Autodesk Fusion 360 part; units mm, degrees
(part 2 of 6)
  arc A437 (-116.0003, -83.2613) -> (-115.4978, -80.8724) centre (-117.2994, -81.7407) ccw
  arc A438 (-109.575, -88.7321) -> (-112.01, -88.5567) centre (-110.9063, -90.2247) ccw
  arc A439 (-112.6799, -88.4476) -> (-112.01, -88.5567) centre (-112.2859, -88.1398) ccw
  line L220 (-112.88, -88.1915) -> (-112.6799, -88.4476)
  line L221 (-112.88, -88.1915) -> (-113.08, -87.9354)
  arc A440 (-113.0239, -87.259) -> (-113.08, -87.9354) centre (-112.686, -87.6276) ccw
  arc A441 (-113.0239, -87.259) -> (-112.605, -84.8539) centre (-114.3753, -85.7846) ccw
  arc A442 (-106.4116, -92.5022) -> (-108.8511, -92.4119) centre (-107.6899, -94.0403) ccw
  arc A443 (-109.5244, -92.3262) -> (-108.8511, -92.4119) centre (-109.1414, -92.0048) ccw
  line L222 (-109.7334, -92.0772) -> (-109.5244, -92.3262)
  line L223 (-109.7334, -92.0772) -> (-109.9423, -91.8283)
  arc A444 (-109.9097, -91.1503) -> (-109.9423, -91.8283) centre (-109.5592, -91.5069) ccw
  arc A445 (-109.9097, -91.1503) -> (-109.575, -88.7321) centre (-111.3118, -89.724) ccw
  arc A446 (-103.1185, -96.1595) -> (-105.5597, -96.1544) centre (-104.3424, -97.7413) ccw
  arc A447 (-106.2356, -96.0923) -> (-105.5597, -96.1544) centre (-105.864, -95.7577) ccw
  line L224 (-106.4531, -95.8508) -> (-106.2356, -96.0923)
  line L225 (-106.4531, -95.8508) -> (-106.6705, -95.6092)
  arc A448 (-106.6617, -94.9306) -> (-106.6705, -95.6092) centre (-106.299, -95.2747) ccw
  arc A449 (-106.6617, -94.9306) -> (-106.4116, -92.5022) centre (-108.1126, -93.554) ccw
  arc A450 (-99.6997, -99.6997) -> (-102.1396, -99.7798) centre (-100.8677, -101.3233) ccw
  arc A451 (-102.8173, -99.7413) -> (-102.1396, -99.7798) centre (-102.4576, -99.394) ccw
  line L226 (-103.0431, -99.5075) -> (-102.8173, -99.7413)
  line L227 (-103.0431, -99.5075) -> (-103.2688, -99.2737)
  arc A452 (-103.2837, -98.5952) -> (-103.2688, -99.2737) centre (-102.9092, -98.9264) ccw
  arc A453 (-103.2837, -98.5952) -> (-103.1185, -96.1595) centre (-104.7818, -97.2701) ccw
  arc A454 (-96.1595, -103.1185) -> (-98.5952, -103.2837) centre (-97.2701, -104.7818) ccw
  arc A455 (-99.2737, -103.2688) -> (-98.5952, -103.2837) centre (-98.9264, -102.9092) ccw
  line L228 (-99.5075, -103.0431) -> (-99.2737, -103.2688)
  line L229 (-99.5075, -103.0431) -> (-99.7413, -102.8173)
  arc A456 (-99.7798, -102.1396) -> (-99.7413, -102.8173) centre (-99.394, -102.4576) ccw
  arc A457 (-99.7798, -102.1396) -> (-99.6997, -99.6997) centre (-101.3233, -100.8677) ccw
  arc A458 (-92.5022, -106.4116) -> (-94.9306, -106.6617) centre (-93.554, -108.1126) ccw
  arc A459 (-95.6092, -106.6705) -> (-94.9306, -106.6617) centre (-95.2747, -106.299) ccw
  line L230 (-95.8508, -106.4531) -> (-95.6092, -106.6705)
  line L231 (-95.8508, -106.4531) -> (-96.0923, -106.2356)
  arc A460 (-96.1544, -105.5597) -> (-96.0923, -106.2356) centre (-95.7577, -105.864) ccw
  arc A461 (-96.1544, -105.5597) -> (-96.1595, -103.1185) centre (-97.7413, -104.3424) ccw
  arc A462 (-88.7321, -109.575) -> (-91.1503, -109.9097) centre (-89.724, -111.3118) ccw
  arc A463 (-91.8283, -109.9423) -> (-91.1503, -109.9097) centre (-91.5069, -109.5592) ccw
  line L232 (-92.0772, -109.7334) -> (-91.8283, -109.9423)
  line L233 (-92.0772, -109.7334) -> (-92.3262, -109.5244)
  arc A464 (-92.4119, -108.8511) -> (-92.3262, -109.5244) centre (-92.0048, -109.1414) ccw
  arc A465 (-92.4119, -108.8511) -> (-92.5022, -106.4116) centre (-94.0403, -107.6899) ccw
  arc A466 (-84.8539, -112.605) -> (-87.259, -113.0239) centre (-85.7846, -114.3753) ccw
  arc A467 (-87.9354, -113.08) -> (-87.259, -113.0239) centre (-87.6276, -112.686) ccw
  line L234 (-88.1915, -112.88) -> (-87.9354, -113.08)
  line L235 (-88.1915, -112.88) -> (-88.4476, -112.6799)
  arc A468 (-88.5567, -112.01) -> (-88.4476, -112.6799) centre (-88.1398, -112.2859) ccw
  arc A469 (-88.5567, -112.01) -> (-88.7321, -109.575) centre (-90.2247, -110.9063) ccw
  arc A470 (-80.8724, -115.4978) -> (-83.2613, -116.0003) centre (-81.7407, -117.2994) ccw
  arc A471 (-83.9354, -116.0801) -> (-83.2613, -116.0003) centre (-83.6415, -115.6756) ccw
  line L236 (-84.1983, -115.889) -> (-83.9354, -116.0801)
  line L237 (-84.1983, -115.889) -> (-84.4612, -115.698)
  arc A472 (-84.5937, -115.0323) -> (-84.4612, -115.698) centre (-84.1673, -115.2935) ccw
  arc A473 (-84.5937, -115.0323) -> (-84.8539, -112.605) centre (-86.2991, -113.9875) ccw
  arc A474 (-76.7923, -118.2498) -> (-79.1623, -118.8354) centre (-77.5972, -120.0807) ccw
  arc A475 (-79.8331, -118.9387) -> (-79.1623, -118.8354) centre (-79.5535, -118.5241) ccw
  line L238 (-80.1025, -118.7569) -> (-79.8331, -118.9387)
  line L239 (-80.1025, -118.7569) -> (-80.372, -118.5752)
  arc A476 (-80.5276, -117.9145) -> (-80.372, -118.5752) centre (-80.0924, -118.1607) ccw
  arc A477 (-80.5276, -117.9145) -> (-80.8724, -115.4978) centre (-82.2684, -116.9299) ccw
  arc A478 (-72.6187, -120.8578) -> (-74.9667, -121.5258) centre (-73.3592, -122.7156) ccw
  arc A479 (-75.6336, -121.6523) -> (-74.9667, -121.5258) centre (-75.3686, -121.2283) ccw
  line L240 (-75.9092, -121.4801) -> (-75.6336, -121.6523)
  line L241 (-75.9092, -121.4801) -> (-76.1848, -121.3079)
  arc A480 (-76.3634, -120.653) -> (-76.1848, -121.3079) centre (-75.9199, -120.8839) ccw
  arc A481 (-76.3634, -120.653) -> (-76.7923, -118.2498) centre (-78.1375, -119.7298) ccw
  arc A482 (-68.3566, -123.3185) -> (-70.6799, -124.068) centre (-69.0318, -125.2011) ccw
  arc A483 (-71.3419, -124.2178) -> (-70.6799, -124.068) centre (-71.0919, -123.7848) ccw
  line L242 (-71.6234, -124.0553) -> (-71.3419, -124.2178)
  line L243 (-71.6234, -124.0553) -> (-71.9048, -123.8928)
  arc A484 (-72.1061, -123.2446) -> (-71.9048, -123.8928) centre (-71.6548, -123.4598) ccw
  arc A485 (-72.1061, -123.2446) -> (-72.6187, -120.8578) centre (-73.9114, -122.3838) ccw
  arc A486 (-64.0112, -125.629) -> (-66.3069, -126.4592) centre (-64.6203, -127.534) ccw
  arc A487 (-66.9633, -126.6319) -> (-66.3069, -126.4592) centre (-66.7286, -126.1905) ccw
  line L244 (-67.2503, -126.4793) -> (-66.9633, -126.6319)
  line L245 (-67.2503, -126.4793) -> (-67.5372, -126.3268)
  arc A488 (-67.761, -125.686) -> (-67.5372, -126.3268) centre (-67.3025, -125.8853) ccw
  arc A489 (-67.761, -125.686) -> (-68.3566, -123.3185) centre (-69.5953, -124.8887) ccw
  arc A490 (-59.5878, -127.7864) -> (-61.8532, -128.6962) centre (-60.13, -129.7115) ccw
  arc A491 (-62.5031, -128.8918) -> (-61.8532, -128.6962) centre (-62.2839, -128.4424) ccw
  line L246 (-62.7952, -128.7493) -> (-62.5031, -128.8918)
  line L247 (-62.7952, -128.7493) -> (-63.0873, -128.6068)
  arc A492 (-63.3334, -127.9742) -> (-63.0873, -128.6068) centre (-62.8682, -128.1574) ccw
  arc A493 (-63.3334, -127.9742) -> (-64.0112, -125.629) centre (-65.1943, -127.2415) ccw
  arc A494 (-55.0918, -129.7882) -> (-57.324, -130.7764) centre (-55.5665, -131.731) ccw
  arc A495 (-57.9668, -130.9946) -> (-57.324, -130.7764) centre (-57.7634, -130.5378) ccw
  line L248 (-58.2637, -130.8624) -> (-57.9668, -130.9946)
  line L249 (-58.2637, -130.8624) -> (-58.5606, -130.7302)
  arc A496 (-58.8286, -130.1066) -> (-58.5606, -130.7302) centre (-58.3572, -130.2734) ccw
  arc A497 (-58.8286, -130.1066) -> (-59.5878, -127.7864) centre (-60.7139, -129.4392) ccw
  arc A498 (-50.5287, -131.6318) -> (-52.7251, -132.6974) centre (-50.9353, -133.59) ccw
  arc A499 (-53.3598, -132.9378) -> (-52.7251, -132.6974) centre (-53.1725, -132.4742) ccw
  line L250 (-53.6612, -132.816) -> (-53.3598, -132.9378)
  line L251 (-53.6612, -132.816) -> (-53.9625, -132.6943)
  arc A500 (-54.2521, -132.0804) -> (-53.9625, -132.6943) centre (-53.7752, -132.2307) ccw
  arc A501 (-54.2521, -132.0804) -> (-55.0918, -129.7882) centre (-56.1596, -131.4793) ccw
  arc A502 (-45.904, -133.315) -> (-48.0619, -134.4566) centre (-46.2421, -135.2862) ccw
  arc A503 (-48.6879, -134.719) -> (-48.0619, -134.4566) centre (-48.5169, -134.2492) ccw
  line L252 (-48.9933, -134.6079) -> (-48.6879, -134.719)
  line L253 (-48.9933, -134.6079) -> (-49.2987, -134.4967)
  arc A504 (-49.6095, -133.8933) -> (-49.2987, -134.4967) centre (-49.1277, -134.0269) ccw
  arc A505 (-49.6095, -133.8933) -> (-50.5287, -131.6318) centre (-51.5368, -133.3591) ccw
  arc A506 (-41.2235, -134.8358) -> (-43.3402, -136.052) centre (-41.4925, -136.8177) ccw
  arc A507 (-43.9566, -136.3362) -> (-43.3402, -136.052) centre (-43.8021, -135.8606) ccw
  line L254 (-44.2657, -136.2357) -> (-43.9566, -136.3362)
  line L255 (-44.2657, -136.2357) -> (-44.5748, -136.1353)
  arc A508 (-44.9065, -135.5431) -> (-44.5748, -136.1353) centre (-44.4203, -135.6598) ccw
  arc A509 (-44.9065, -135.5431) -> (-45.904, -133.315) centre (-46.8513, -135.0765) ccw
  arc A510 (-36.4926, -136.1924) -> (-38.5656, -137.4817) centre (-36.6924, -138.1824) ccw
  arc A511 (-39.1717, -137.7872) -> (-38.5656, -137.4817) centre (-39.0339, -137.3065) ccw
  line L256 (-39.4841, -137.6976) -> (-39.1717, -137.7872)
  line L257 (-39.4841, -137.6976) -> (-39.7966, -137.608)
  arc A512 (-40.1487, -137.0278) -> (-39.7966, -137.608) centre (-39.6587, -137.1274) ccw
  arc A513 (-40.1487, -137.0278) -> (-41.2235, -134.8358) centre (-42.1086, -136.6293) ccw
  arc A514 (-31.7174, -137.383) -> (-33.7441, -138.7439) centre (-31.8475, -139.3787) ccw
  arc A515 (-34.3392, -139.0703) -> (-33.7441, -138.7439) centre (-34.2182, -138.5852) ccw
  line L258 (-34.6545, -138.9917) -> (-34.3392, -139.0703)
  line L259 (-34.6545, -138.9917) -> (-34.9699, -138.9131)
  arc A516 (-35.3421, -138.3455) -> (-34.9699, -138.9131) centre (-34.8489, -138.4279) ccw
  arc A517 (-35.3421, -138.3455) -> (-36.4926, -136.1924) centre (-37.3147, -138.0156) ccw
  arc A518 (-26.9034, -138.4062) -> (-28.8814, -139.837) centre (-26.9639, -140.4053) ccw
  arc A519 (-29.4648, -140.184) -> (-28.8814, -139.837) centre (-29.3608, -139.6949) ccw
  line L260 (-29.7827, -140.1164) -> (-29.4648, -140.184)
  line L261 (-29.7827, -140.1164) -> (-30.1006, -140.0489)
  arc A520 (-30.4923, -139.4946) -> (-30.1006, -140.0489) centre (-29.9966, -139.5598) ccw
  arc A521 (-30.4923, -139.4946) -> (-31.7174, -137.383) centre (-32.4753, -139.2338) ccw
  arc A522 (-22.0567, -139.2608) -> (-23.9836, -140.7598) centre (-22.0474, -141.2608) ccw
  arc A523 (-24.5545, -141.1269) -> (-23.9836, -140.7598) centre (-24.4676, -140.6345) ccw
  line L262 (-24.8745, -141.0705) -> (-24.5545, -141.1269)
  line L263 (-24.8745, -141.0705) -> (-25.1946, -141.014)
  arc A524 (-25.6055, -140.4738) -> (-25.1946, -141.014) centre (-25.1078, -140.5216) ccw
  arc A525 (-25.6055, -140.4738) -> (-26.9034, -138.4062) centre (-27.5963, -140.2824) ccw
  arc A526 (-17.1832, -139.9458) -> (-19.0565, -141.511) centre (-17.104, -141.9442) ccw
  arc A527 (-19.6143, -141.8979) -> (-19.0565, -141.511) centre (-19.5447, -141.4028) ccw
  line L264 (-19.9361, -141.8527) -> (-19.6143, -141.8979)
  line L265 (-19.9361, -141.8527) -> (-20.2579, -141.8074)
  arc A528 (-20.6874, -141.2818) -> (-20.2579, -141.8074) centre (-20.1883, -141.3123) ccw
  arc A529 (-20.6874, -141.2818) -> (-22.0567, -139.2608) centre (-22.6837, -141.16) ccw
  arc A530 (-12.2887, -140.4602) -> (-14.1063, -142.0899) centre (-12.1398, -142.4546) ccw
  arc A531 (-14.6501, -142.496) -> (-14.1063, -142.0899) centre (-14.5979, -141.9987) ccw
  line L266 (-14.9734, -142.462) -> (-14.6501, -142.496)
  line L267 (-14.9734, -142.462) -> (-15.2966, -142.428)
  arc A532 (-15.7441, -141.9177) -> (-15.2966, -142.428) centre (-15.2443, -141.9308) ccw
  arc A533 (-15.7441, -141.9177) -> (-17.1832, -139.9458) centre (-17.7435, -141.8657) ccw
  arc A534 (-7.3792, -140.8035) -> (-9.1388, -142.4956) centre (-7.1608, -142.7915) ccw
  arc A535 (-9.6682, -142.9205) -> (-9.1388, -142.4956) centre (-9.6333, -142.4217) ccw
  line L268 (-9.9924, -142.8978) -> (-9.6682, -142.9205)
  line L269 (-9.9924, -142.8978) -> (-10.3166, -142.8751)
  arc A536 (-10.7817, -142.3808) -> (-10.3166, -142.8751) centre (-10.2817, -142.3763) ccw
  arc A537 (-10.7817, -142.3808) -> (-12.2887, -140.4602) centre (-12.7816, -142.3985) ccw
  arc A538 (-2.4607, -140.9752) -> (-4.1602, -142.7278) centre (-2.1731, -142.9545) ccw
  arc A539 (-4.6744, -143.1708) -> (-4.1602, -142.7278) centre (-4.657, -142.6711) ccw
  line L270 (-4.9992, -143.1595) -> (-4.6744, -143.1708)
  line L271 (-4.9992, -143.1595) -> (-5.324, -143.1481)
  arc A540 (-5.8061, -142.6703) -> (-5.324, -143.1481) centre (-5.3066, -142.6484) ccw
  arc A541 (-5.8061, -142.6703) -> (-7.3792, -140.8035) centre (-7.8042, -142.7578) ccw
  arc A542 (2.4607, -140.9752) -> (0.8235, -142.786) centre (2.8173, -142.9432) ccw
  arc A543 (0.325, -143.2467) -> (0.8235, -142.786) centre (0.325, -142.7467) ccw
  line L272 (0, -143.2467) -> (0.325, -143.2467)
  line L273 (0, -143.2467) -> (-0.325, -143.2467)
  arc A544 (-0.8235, -142.786) -> (-0.325, -143.2467) centre (-0.325, -142.7467) ccw
  arc A545 (-0.8235, -142.786) -> (-2.4607, -140.9752) centre (-2.8173, -142.9432) ccw
  arc A546 (7.3792, -140.8035) -> (5.8061, -142.6703) centre (7.8042, -142.7578) ccw
  arc A547 (5.324, -143.1481) -> (5.8061, -142.6703) centre (5.3066, -142.6484) ccw
  line L274 (4.9992, -143.1595) -> (5.324, -143.1481)
  line L275 (4.9992, -143.1595) -> (4.6744, -143.1708)
  arc A548 (4.1602, -142.7278) -> (4.6744, -143.1708) centre (4.657, -142.6711) ccw
  arc A549 (4.1602, -142.7278) -> (2.4607, -140.9752) centre (2.1731, -142.9545) ccw
  arc A550 (12.2887, -140.4602) -> (10.7817, -142.3808) centre (12.7816, -142.3985) ccw
  arc A551 (10.3166, -142.8751) -> (10.7817, -142.3808) centre (10.2817, -142.3763) ccw
  line L276 (9.9924, -142.8978) -> (10.3166, -142.8751)
  line L277 (9.9924, -142.8978) -> (9.6682, -142.9205)
  arc A552 (9.1388, -142.4956) -> (9.6682, -142.9205) centre (9.6333, -142.4217) ccw
  arc A553 (9.1388, -142.4956) -> (7.3792, -140.8035) centre (7.1608, -142.7915) ccw
  arc A554 (17.1832, -139.9458) -> (15.7441, -141.9177) centre (17.7435, -141.8657) ccw
  arc A555 (15.2966, -142.428) -> (15.7441, -141.9177) centre (15.2443, -141.9308) ccw
  line L278 (14.9734, -142.462) -> (15.2966, -142.428)
  line L279 (14.9734, -142.462) -> (14.6501, -142.496)
  arc A556 (14.1063, -142.0899) -> (14.6501, -142.496) centre (14.5979, -141.9987) ccw
  arc A557 (14.1063, -142.0899) -> (12.2887, -140.4602) centre (12.1398, -142.4546) ccw
  arc A558 (22.0567, -139.2608) -> (20.6874, -141.2818) centre (22.6837, -141.16) ccw
  arc A559 (20.2579, -141.8074) -> (20.6874, -141.2818) centre (20.1883, -141.3123) ccw
  line L280 (19.9361, -141.8527) -> (20.2579, -141.8074)
  line L281 (19.9361, -141.8527) -> (19.6143, -141.8979)
  arc A560 (19.0565, -141.511) -> (19.6143, -141.8979) centre (19.5447, -141.4028) ccw
  arc A561 (19.0565, -141.511) -> (17.1832, -139.9458) centre (17.104, -141.9442) ccw
  arc A562 (26.9034, -138.4062) -> (25.6055, -140.4738) centre (27.5963, -140.2824) ccw
  arc A563 (25.1946, -141.014) -> (25.6055, -140.4738) centre (25.1078, -140.5216) ccw
  line L282 (24.8745, -141.0705) -> (25.1946, -141.014)
  line L283 (24.8745, -141.0705) -> (24.5545, -141.1269)
  arc A564 (23.9836, -140.7598) -> (24.5545, -141.1269) centre (24.4676, -140.6345) ccw
  arc A565 (23.9836, -140.7598) -> (22.0567, -139.2608) centre (22.0474, -141.2608) ccw
  arc A566 (31.7174, -137.383) -> (30.4923, -139.4946) centre (32.4753, -139.2338) ccw
  arc A567 (30.1006, -140.0489) -> (30.4923, -139.4946) centre (29.9966, -139.5598) ccw
  line L284 (29.7827, -140.1164) -> (30.1006, -140.0489)
  line L285 (29.7827, -140.1164) -> (29.4648, -140.184)
  arc A568 (28.8814, -139.837) -> (29.4648, -140.184) centre (29.3608, -139.6949) ccw
  arc A569 (28.8814, -139.837) -> (26.9034, -138.4062) centre (26.9639, -140.4053) ccw
  arc A570 (36.4926, -136.1924) -> (35.3421, -138.3455) centre (37.3147, -138.0156) ccw
  arc A571 (34.9699, -138.9131) -> (35.3421, -138.3455) centre (34.8489, -138.4279) ccw
  line L286 (34.6545, -138.9917) -> (34.9699, -138.9131)
  line L287 (34.6545, -138.9917) -> (34.3392, -139.0703)
  arc A572 (33.7441, -138.7439) -> (34.3392, -139.0703) centre (34.2182, -138.5852) ccw
  arc A573 (33.7441, -138.7439) -> (31.7174, -137.383) centre (31.8475, -139.3787) ccw
  arc A574 (41.2235, -134.8358) -> (40.1487, -137.0278) centre (42.1086, -136.6293) ccw
  arc A575 (39.7966, -137.608) -> (40.1487, -137.0278) centre (39.6587, -137.1274) ccw
  line L288 (39.4841, -137.6976) -> (39.7966, -137.608)
  line L289 (39.4841, -137.6976) -> (39.1717, -137.7872)
  arc A576 (38.5656, -137.4817) -> (39.1717, -137.7872) centre (39.0339, -137.3065) ccw
  arc A577 (38.5656, -137.4817) -> (36.4926, -136.1924) centre (36.6924, -138.1824) ccw
  arc A578 (45.904, -133.315) -> (44.9065, -135.5431) centre (46.8513, -135.0765) ccw
  arc A579 (44.5748, -136.1353) -> (44.9065, -135.5431) centre (44.4203, -135.6598) ccw
  line L290 (44.2657, -136.2357) -> (44.5748, -136.1353)
  line L291 (44.2657, -136.2357) -> (43.9566, -136.3362)
  arc A580 (43.3402, -136.052) -> (43.9566, -136.3362) centre (43.8021, -135.8606) ccw
  arc A581 (43.3402, -136.052) -> (41.2235, -134.8358) centre (41.4925, -136.8177) ccw
  arc A582 (50.5287, -131.6318) -> (49.6095, -133.8933) centre (51.5368, -133.3591) ccw
  arc A583 (49.2987, -134.4967) -> (49.6095, -133.8933) centre (49.1277, -134.0269) ccw
  line L292 (48.9933, -134.6079) -> (49.2987, -134.4967)
  line L293 (48.9933, -134.6079) -> (48.6879, -134.719)
  arc A584 (48.0619, -134.4566) -> (48.6879, -134.719) centre (48.5169, -134.2492) ccw
  arc A585 (48.0619, -134.4566) -> (45.904, -133.315) centre (46.2421, -135.2862) ccw
  arc A586 (55.0918, -129.7882) -> (54.2521, -132.0804) centre (56.1596, -131.4793) ccw
  arc A587 (53.9625, -132.6943) -> (54.2521, -132.0804) centre (53.7752, -132.2307) ccw
  line L294 (53.6612, -132.816) -> (53.9625, -132.6943)
  line L295 (53.6612, -132.816) -> (53.3598, -132.9378)
  arc A588 (52.7251, -132.6974) -> (53.3598, -132.9378) centre (53.1725, -132.4742) ccw
  arc A589 (52.7251, -132.6974) -> (50.5287, -131.6318) centre (50.9353, -133.59) ccw
  arc A590 (59.5878, -127.7864) -> (58.8286, -130.1066) centre (60.7139, -129.4392) ccw
  arc A591 (58.5606, -130.7302) -> (58.8286, -130.1066) centre (58.3572, -130.2734) ccw
  line L296 (58.2637, -130.8624) -> (58.5606, -130.7302)
  line L297 (58.2637, -130.8624) -> (57.9668, -130.9946)
  arc A592 (57.324, -130.7764) -> (57.9668, -130.9946) centre (57.7634, -130.5378) ccw
  arc A593 (57.324, -130.7764) -> (55.0918, -129.7882) centre (55.5665, -131.731) ccw
  arc A594 (64.0112, -125.629) -> (63.3334, -127.9742) centre (65.1943, -127.2415) ccw
  arc A595 (63.0873, -128.6068) -> (63.3334, -127.9742) centre (62.8682, -128.1574) ccw
  line L298 (62.7952, -128.7493) -> (63.0873, -128.6068)
  line L299 (62.7952, -128.7493) -> (62.5031, -128.8918)
  arc A596 (61.8532, -128.6962) -> (62.5031, -128.8918) centre (62.2839, -128.4424) ccw
  arc A597 (61.8532, -128.6962) -> (59.5878, -127.7864) centre (60.13, -129.7115) ccw
  arc A598 (68.3566, -123.3185) -> (67.761, -125.686) centre (69.5953, -124.8887) ccw
  arc A599 (67.5372, -126.3268) -> (67.761, -125.686) centre (67.3025, -125.8853) ccw
  line L300 (67.2503, -126.4793) -> (67.5372, -126.3268)
  line L301 (67.2503, -126.4793) -> (66.9633, -126.6319)
  arc A600 (66.3069, -126.4592) -> (66.9633, -126.6319) centre (66.7286, -126.1905) ccw
  arc A601 (66.3069, -126.4592) -> (64.0112, -125.629) centre (64.6203, -127.534) ccw
  arc A602 (72.6187, -120.8578) -> (72.1061, -123.2446) centre (73.9114, -122.3838) ccw
  arc A603 (71.9048, -123.8928) -> (72.1061, -123.2446) centre (71.6548, -123.4598) ccw
  line L302 (71.6234, -124.0553) -> (71.9048, -123.8928)
  line L303 (71.6234, -124.0553) -> (71.3419, -124.2178)
  arc A604 (70.6799, -124.068) -> (71.3419, -124.2178) centre (71.0919, -123.7848) ccw
  arc A605 (70.6799, -124.068) -> (68.3566, -123.3185) centre (69.0318, -125.2011) ccw
  arc A606 (76.7923, -118.2498) -> (76.3634, -120.653) centre (78.1375, -119.7298) ccw
  arc A607 (76.1848, -121.3079) -> (76.3634, -120.653) centre (75.9199, -120.8839) ccw
  line L304 (75.9092, -121.4801) -> (76.1848, -121.3079)
  line L305 (75.9092, -121.4801) -> (75.6336, -121.6523)
  arc A608 (74.9667, -121.5258) -> (75.6336, -121.6523) centre (75.3686, -121.2283) ccw
  arc A609 (74.9667, -121.5258) -> (72.6187, -120.8578) centre (73.3592, -122.7156) ccw
  arc A610 (80.8724, -115.4978) -> (80.5276, -117.9145) centre (82.2684, -116.9299) ccw
  arc A611 (80.372, -118.5752) -> (80.5276, -117.9145) centre (80.0924, -118.1607) ccw
  line L306 (80.1025, -118.7569) -> (80.372, -118.5752)
  line L307 (80.1025, -118.7569) -> (79.8331, -118.9387)
  arc A612 (79.1623, -118.8354) -> (79.8331, -118.9387) centre (79.5535, -118.5241) ccw
  arc A613 (79.1623, -118.8354) -> (76.7923, -118.2498) centre (77.5972, -120.0807) ccw
  arc A614 (84.8539, -112.605) -> (84.5937, -115.0323) centre (86.2991, -113.9875) ccw
  arc A615 (84.4612, -115.698) -> (84.5937, -115.0323) centre (84.1673, -115.2935) ccw
  line L308 (84.1983, -115.889) -> (84.4612, -115.698)
  line L309 (84.1983, -115.889) -> (83.9354, -116.0801)
  arc A616 (83.2613, -116.0003) -> (83.9354, -116.0801) centre (83.6415, -115.6756) ccw
  arc A617 (83.2613, -116.0003) -> (80.8724, -115.4978) centre (81.7407, -117.2994) ccw
  arc A618 (88.7321, -109.575) -> (88.5567, -112.01) centre (90.2247, -110.9063) ccw
  arc A619 (88.4476, -112.6799) -> (88.5567, -112.01) centre (88.1398, -112.2859) ccw
  line L310 (88.1915, -112.88) -> (88.4476, -112.6799)
  line L311 (88.1915, -112.88) -> (87.9354, -113.08)
  arc A620 (87.259, -113.0239) -> (87.9354, -113.08) centre (87.6276, -112.686) ccw
  arc A621 (87.259, -113.0239) -> (84.8539, -112.605) centre (85.7846, -114.3753) ccw
  arc A622 (92.5022, -106.4116) -> (92.4119, -108.8511) centre (94.0403, -107.6899) ccw
  arc A623 (92.3262, -109.5244) -> (92.4119, -108.8511) centre (92.0048, -109.1414) ccw
  line L312 (92.0772, -109.7334) -> (92.3262, -109.5244)
  line L313 (92.0772, -109.7334) -> (91.8283, -109.9423)
  arc A624 (91.1503, -109.9097) -> (91.8283, -109.9423) centre (91.5069, -109.5592) ccw
  arc A625 (91.1503, -109.9097) -> (88.7321, -109.575) centre (89.724, -111.3118) ccw
  arc A626 (96.1595, -103.1185) -> (96.1544, -105.5597) centre (97.7413, -104.3424) ccw
  arc A627 (96.0923, -106.2356) -> (96.1544, -105.5597) centre (95.7577, -105.864) ccw
  line L314 (95.8508, -106.4531) -> (96.0923, -106.2356)
  line L315 (95.8508, -106.4531) -> (95.6092, -106.6705)
  arc A628 (94.9306, -106.6617) -> (95.6092, -106.6705) centre (95.2747, -106.299) ccw
  arc A629 (94.9306, -106.6617) -> (92.5022, -106.4116) centre (93.554, -108.1126) ccw
  arc A630 (99.6997, -99.6997) -> (99.7798, -102.1396) centre (101.3233, -100.8677) ccw
  arc A631 (99.7413, -102.8173) -> (99.7798, -102.1396) centre (99.394, -102.4576) ccw
  line L316 (99.5075, -103.0431) -> (99.7413, -102.8173)
  line L317 (99.5075, -103.0431) -> (99.2737, -103.2688)
  arc A632 (98.5952, -103.2837) -> (99.2737, -103.2688) centre (98.9264, -102.9092) ccw
  arc A633 (98.5952, -103.2837) -> (96.1595, -103.1185) centre (97.2701, -104.7818) ccw
  arc A634 (103.1185, -96.1595) -> (103.2837, -98.5952) centre (104.7818, -97.2701) ccw
  arc A635 (103.2688, -99.2737) -> (103.2837, -98.5952) centre (102.9092, -98.9264) ccw
  line L318 (103.0431, -99.5075) -> (103.2688, -99.2737)
  line L319 (103.0431, -99.5075) -> (102.8173, -99.7413)
  arc A636 (102.1396, -99.7798) -> (102.8173, -99.7413) centre (102.4576, -99.394) ccw
  arc A637 (102.1396, -99.7798) -> (99.6997, -99.6997) centre (100.8677, -101.3233) ccw
  arc A638 (106.4116, -92.5022) -> (106.6617, -94.9306) centre (108.1126, -93.554) ccw
  arc A639 (106.6705, -95.6092) -> (106.6617, -94.9306) centre (106.299, -95.2747) ccw
  line L320 (106.4531, -95.8508) -> (106.6705, -95.6092)
  line L321 (106.4531, -95.8508) -> (106.2356, -96.0923)
  arc A640 (105.5597, -96.1544) -> (106.2356, -96.0923) centre (105.864, -95.7577) ccw
  arc A641 (105.5597, -96.1544) -> (103.1185, -96.1595) centre (104.3424, -97.7413) ccw
  arc A642 (109.575, -88.7321) -> (109.9097, -91.1503) centre (111.3118, -89.724) ccw
  arc A643 (109.9423, -91.8283) -> (109.9097, -91.1503) centre (109.5592, -91.5069) ccw
  line L322 (109.7334, -92.0772) -> (109.9423, -91.8283)
  line L323 (109.7334, -92.0772) -> (109.5244, -92.3262)
  arc A644 (108.8511, -92.4119) -> (109.5244, -92.3262) centre (109.1414, -92.0048) ccw
  arc A645 (108.8511, -92.4119) -> (106.4116, -92.5022) centre (107.6899, -94.0403) ccw
  arc A646 (112.605, -84.8539) -> (113.0239, -87.259) centre (114.3753, -85.7846) ccw
  arc A647 (113.08, -87.9354) -> (113.0239, -87.259) centre (112.686, -87.6276) ccw
  line L324 (112.88, -88.1915) -> (113.08, -87.9354)
  line L325 (112.88, -88.1915) -> (112.6799, -88.4476)
  arc A648 (112.01, -88.5567) -> (112.6799, -88.4476) centre (112.2859, -88.1398) ccw
  arc A649 (112.01, -88.5567) -> (109.575, -88.7321) centre (110.9063, -90.2247) ccw
  arc A650 (115.4978, -80.8724) -> (116.0003, -83.2613) centre (117.2994, -81.7407) ccw
  arc A651 (116.0801, -83.9354) -> (116.0003, -83.2613) centre (115.6756, -83.6415) ccw
  line L326 (115.889, -84.1983) -> (116.0801, -83.9354)
  line L327 (115.889, -84.1983) -> (115.698, -84.4612)
  arc A652 (115.0323, -84.5937) -> (115.698, -84.4612) centre (115.2935, -84.1673) ccw
  arc A653 (115.0323, -84.5937) -> (112.605, -84.8539) centre (113.9875, -86.2991) ccw
  arc A654 (118.2498, -76.7923) -> (118.8354, -79.1623) centre (120.0807, -77.5972) ccw
  arc A655 (118.9387, -79.8331) -> (118.8354, -79.1623) centre (118.5241, -79.5535) ccw
  line L328 (118.7569, -80.1025) -> (118.9387, -79.8331)
  line L329 (118.7569, -80.1025) -> (118.5752, -80.372)
  arc A656 (117.9145, -80.5276) -> (118.5752, -80.372) centre (118.1607, -80.0924) ccw
  arc A657 (117.9145, -80.5276) -> (115.4978, -80.8724) centre (116.9299, -82.2684) ccw
  arc A658 (120.8578, -72.6187) -> (121.5258, -74.9667) centre (122.7156, -73.3592) ccw
  arc A659 (121.6523, -75.6336) -> (121.5258, -74.9667) centre (121.2283, -75.3686) ccw
  line L330 (121.4801, -75.9092) -> (121.6523, -75.6336)
  line L331 (121.4801, -75.9092) -> (121.3079, -76.1848)
  arc A660 (120.653, -76.3634) -> (121.3079, -76.1848) centre (120.8839, -75.9199) ccw
  arc A661 (120.653, -76.3634) -> (118.2498, -76.7923) centre (119.7298, -78.1375) ccw
  arc A662 (123.3185, -68.3566) -> (124.068, -70.6799) centre (125.2011, -69.0318) ccw
  arc A663 (124.2178, -71.3419) -> (124.068, -70.6799) centre (123.7848, -71.0919) ccw
  line L332 (124.0553, -71.6234) -> (124.2178, -71.3419)
  line L333 (124.0553, -71.6234) -> (123.8928, -71.9048)
  arc A664 (123.2446, -72.1061) -> (123.8928, -71.9048) centre (123.4598, -71.6548) ccw
  arc A665 (123.2446, -72.1061) -> (120.8578, -72.6187) centre (122.3838, -73.9114) ccw
  arc A666 (125.629, -64.0112) -> (126.4592, -66.3069) centre (127.534, -64.6203) ccw
  arc A667 (126.6319, -66.9633) -> (126.4592, -66.3069) centre (126.1905, -66.7286) ccw
  line L334 (126.4793, -67.2503) -> (126.6319, -66.9633)
  line L335 (126.4793, -67.2503) -> (126.3268, -67.5372)
  arc A668 (125.686, -67.761) -> (126.3268, -67.5372) centre (125.8853, -67.3025) ccw
  arc A669 (125.686, -67.761) -> (123.3185, -68.3566) centre (124.8887, -69.5953) ccw
  arc A670 (127.7864, -59.5878) -> (128.6962, -61.8532) centre (129.7115, -60.13) ccw
  arc A671 (128.8918, -62.5031) -> (128.6962, -61.8532) centre (128.4424, -62.2839) ccw
  line L336 (128.7493, -62.7952) -> (128.8918, -62.5031)
  line L337 (128.7493, -62.7952) -> (128.6068, -63.0873)
  arc A672 (127.9742, -63.3334) -> (128.6068, -63.0873) centre (128.1574, -62.8682) ccw
  arc A673 (127.9742, -63.3334) -> (125.629, -64.0112) centre (127.2415, -65.1943) ccw
  arc A674 (129.7882, -55.0918) -> (130.7764, -57.324) centre (131.731, -55.5665) ccw
  arc A675 (130.9946, -57.9668) -> (130.7764, -57.324) centre (130.5378, -57.7634) ccw
  line L338 (130.8624, -58.2637) -> (130.9946, -57.9668)
  line L339 (130.8624, -58.2637) -> (130.7302, -58.5606)
  arc A676 (130.1066, -58.8286) -> (130.7302, -58.5606) centre (130.2734, -58.3572) ccw
  arc A677 (130.1066, -58.8286) -> (127.7864, -59.5878) centre (129.4392, -60.7139) ccw
  arc A678 (131.6318, -50.5287) -> (132.6974, -52.7251) centre (133.59, -50.9353) ccw
  arc A679 (132.9378, -53.3598) -> (132.6974, -52.7251) centre (132.4742, -53.1725) ccw
  line L340 (132.816, -53.6612) -> (132.9378, -53.3598)
  line L341 (132.816, -53.6612) -> (132.6943, -53.9625)
  arc A680 (132.0804, -54.2521) -> (132.6943, -53.9625) centre (132.2307, -53.7752) ccw
  arc A681 (132.0804, -54.2521) -> (129.7882, -55.0918) centre (131.4793, -56.1596) ccw
  arc A682 (133.315, -45.904) -> (134.4566, -48.0619) centre (135.2862, -46.2421) ccw
  arc A683 (134.719, -48.6879) -> (134.4566, -48.0619) centre (134.2492, -48.5169) ccw
  line L342 (134.6079, -48.9933) -> (134.719, -48.6879)
  line L343 (134.6079, -48.9933) -> (134.4967, -49.2987)
  arc A684 (133.8933, -49.6095) -> (134.4967, -49.2987) centre (134.0269, -49.1277) ccw
  arc A685 (133.8933, -49.6095) -> (131.6318, -50.5287) centre (133.3591, -51.5368) ccw
  arc A686 (134.8358, -41.2235) -> (136.052, -43.3402) centre (136.8177, -41.4925) ccw
  arc A687 (136.3362, -43.9566) -> (136.052, -43.3402) centre (135.8606, -43.8021) ccw
  line L344 (136.2357, -44.2657) -> (136.3362, -43.9566)
  line L345 (136.2357, -44.2657) -> (136.1353, -44.5748)
  arc A688 (135.5431, -44.9065) -> (136.1353, -44.5748) centre (135.6598, -44.4203) ccw
  arc A689 (135.5431, -44.9065) -> (133.315, -45.904) centre (135.0765, -46.8513) ccw
  arc A690 (136.1924, -36.4926) -> (137.4817, -38.5656) centre (138.1824, -36.6924) ccw
  arc A691 (137.7872, -39.1717) -> (137.4817, -38.5656) centre (137.3065, -39.0339) ccw
  line L346 (137.6976, -39.4841) -> (137.7872, -39.1717)
  line L347 (137.6976, -39.4841) -> (137.608, -39.7966)
  arc A692 (137.0278, -40.1487) -> (137.608, -39.7966) centre (137.1274, -39.6587) ccw
  arc A693 (137.0278, -40.1487) -> (134.8358, -41.2235) centre (136.6293, -42.1086) ccw
  arc A694 (137.383, -31.7174) -> (138.7439, -33.7441) centre (139.3787, -31.8475) ccw
  arc A695 (139.0703, -34.3392) -> (138.7439, -33.7441) centre (138.5852, -34.2182) ccw
  line L348 (138.9917, -34.6545) -> (139.0703, -34.3392)
  line L349 (138.9917, -34.6545) -> (138.9131, -34.9699)
  arc A696 (138.3455, -35.3421) -> (138.9131, -34.9699) centre (138.4279, -34.8489) ccw
  arc A697 (138.3455, -35.3421) -> (136.1924, -36.4926) centre (138.0156, -37.3147) ccw
  arc A698 (138.4062, -26.9034) -> (139.837, -28.8814) centre (140.4053, -26.9639) ccw
  arc A699 (140.184, -29.4648) -> (139.837, -28.8814) centre (139.6949, -29.3608) ccw
  line L350 (140.1164, -29.7827) -> (140.184, -29.4648)
  line L351 (140.1164, -29.7827) -> (140.0489, -30.1006)
  arc A700 (139.4946, -30.4923) -> (140.0489, -30.1006) centre (139.5598, -29.9966) ccw
  arc A701 (139.4946, -30.4923) -> (137.383, -31.7174) centre (139.2338, -32.4753) ccw
  arc A702 (139.2608, -22.0567) -> (140.7598, -23.9836) centre (141.2608, -22.0474) ccw
  arc A703 (141.1269, -24.5545) -> (140.7598, -23.9836) centre (140.6345, -24.4676) ccw
  line L352 (141.0705, -24.8745) -> (141.1269, -24.5545)
  line L353 (141.0705, -24.8745) -> (141.014, -25.1946)
  arc A704 (140.4738, -25.6055) -> (141.014, -25.1946) centre (140.5216, -25.1078) ccw
  arc A705 (140.4738, -25.6055) -> (138.4062, -26.9034) centre (140.2824, -27.5963) ccw
  arc A706 (139.9458, -17.1832) -> (141.511, -19.0565) centre (141.9442, -17.104) ccw
  arc A707 (141.8979, -19.6143) -> (141.511, -19.0565) centre (141.4028, -19.5447) ccw
  line L354 (141.8527, -19.9361) -> (141.8979, -19.6143)
  line L355 (141.8527, -19.9361) -> (141.8074, -20.2579)
  arc A708 (141.2818, -20.6874) -> (141.8074, -20.2579) centre (141.3123, -20.1883) ccw
  arc A709 (141.2818, -20.6874) -> (139.2608, -22.0567) centre (141.16, -22.6837) ccw
  arc A710 (140.4602, -12.2887) -> (142.0899, -14.1063) centre (142.4546, -12.1398) ccw
  arc A711 (142.496, -14.6501) -> (142.0899, -14.1063) centre (141.9987, -14.5979) ccw
  line L356 (142.462, -14.9734) -> (142.496, -14.6501)
  line L357 (142.462, -14.9734) -> (142.428, -15.2966)
  arc A712 (141.9177, -15.7441) -> (142.428, -15.2966) centre (141.9308, -15.2443) ccw
  arc A713 (141.9177, -15.7441) -> (139.9458, -17.1832) centre (141.8657, -17.7435) ccw
  arc A714 (140.8035, -7.3792) -> (142.4956, -9.1388) centre (142.7915, -7.1608) ccw
  arc A715 (142.9205, -9.6682) -> (142.4956, -9.1388) centre (142.4217, -9.6333) ccw
  line L358 (142.8978, -9.9924) -> (142.9205, -9.6682)
  line L359 (142.8978, -9.9924) -> (142.8751, -10.3166)
  arc A716 (142.3808, -10.7817) -> (142.8751, -10.3166) centre (142.3763, -10.2817) ccw
  arc A717 (142.3808, -10.7817) -> (140.4602, -12.2887) centre (142.3985, -12.7816) ccw
  arc A718 (140.9752, -2.4607) -> (142.7278, -4.1602) centre (142.9545, -2.1731) ccw
  arc A719 (143.1708, -4.6744) -> (142.7278, -4.1602) centre (142.6711, -4.657) ccw
  line L360 (143.1595, -4.9992) -> (143.1708, -4.6744)
  line L361 (143.1595, -4.9992) -> (143.1481, -5.324)
  arc A720 (142.6703, -5.8061) -> (143.1481, -5.324) centre (142.6484, -5.3066) ccw
  arc A721 (142.6703, -5.8061) -> (140.8035, -7.3792) centre (142.7578, -7.8042) ccw
  dimension "d1" = 2.25
  dimension "d2" = 0.5
  dimension "d4" = 0.325
  dimension "d5" = 2
  dimension "d6" = 2.5
  dimension "d7" = 1
  dimension "d9" = 360
  constraint coincident A0.centre A1.centre
  constraint coincident A1 L0.end
  constraint horizontal L0
  constraint coincident A1 L1.end
  constraint vertical L2
  constraint tangent L2 A2
  constraint tangent A2 A3
  constraint coincident A0 A3.start
  constraint coincident L1 A3.start
  constraint symmetric L2.start L0 L3.start
  constraint symmetric L0 L2.end A5.end
  constraint symmetric L0 A2.end A4.start
  constraint symmetric L0 A2 A5
  constraint symmetric L0 A3.start A4.end
  constraint symmetric L0 A3 A4
  measures "d1" distance of A0 A1
  measures "d2" radius of A2
  measures "d4" distance of L0.end L2.end
  measures "d5" radius of A3
  measures "d6" vertical distance of L0.end L1.end
  measures "d7" angle of L0 L1
extrude "Extrude1" add sketch "Sketch1" along normal blind 16